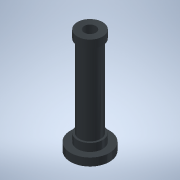
# Autodesk Inventor part: steering_stand_off_bush
Saved by Autodesk Inventor 2020 (Build 240168000, 168)
## iProperties
Created: 2015-12-07
Part Number: steering_stand_off_bush
Material: Hierro, gris
Document SubType Name: Modeling
Designer: MIGUEL ANGEL
Density: 7.15 g/cm^3
Appearance: Gris hierro
Author: MIGUEL ANGEL
Autodesk Inventor part; units mm, degrees
ref_plane "YZ Plane" through (0, 0, 0) normal (1, 0, 0) x (0, 1, 0)
ref_plane "XZ Plane" through (0, 0, 0) normal (0, 1, 0) x (-1, 0, 0)
ref_plane "XY Plane" through (0, 0, 0) normal (0, 0, 1) x (1, 0, 0)
sketch "Boceto1" plane through (0, 0, 0) normal (0, 0, 1) x (1, 0, 0)
  circle A0 centre (0, 0) radius 10
  dimension "d0" = 20
  constraints: 1 centre point, 1 coincident
  measures "d0" diameter of A0
extrude "Extrusión1" add sketch "Boceto1" along normal blind 4
sketch "Boceto2" plane through (0, 0, 4) normal (0, 0, 1) x (1, 0, 0)
  circle A0 centre (0, 0) radius 6.5
  dimension "d3" = 13
  constraints: 1 centre point, 1 coincident
  measures "d3" diameter of A0
extrude "Extrusión2" add sketch "Boceto2" along normal blind 50
sketch "Boceto3" plane through (0, 0, 0) normal (0, 1, 0) x (-1, 0, 0)
  line L0 (6.5, 50) -> (5.5, 50)
  line L1 (5.5, 50) -> (5.5, 8)
  line L2 (5.5, 8) -> (6.5, 8)
  line L3 (0, 30.7495) -> (0, -2.427)
  line L4 (10, 4) -> (-10, 4) projected
  line L5 (6.5, 4) -> (6.5, 54) projected
  point P0 (0, 0)
  dimension "d6" = 1
  dimension "d7" = 4
  dimension "d8" = 4
  constraints: 8 end point, 2 perpendicular, 2 point on line, 1 horizontal, 1 other
  measures "d6" distance of L0.start L0.end
  measures "d7" distance of L5.end L0.start
  measures "d8" distance of L5.start L2.end
revolve "Revolución1" cut sketch "Boceto3" angle 360 about axis through (0, 0, 30.7495) along (0, 0, -1)
sketch "Boceto4" plane through (0, 0, 54) normal (0, 0, 1) x (1, 0, 0)
  circle A0 centre (0, 0) radius 3
  dimension "d10" = 6
  constraints: 1 centre point, 1 coincident
  measures "d10" diameter of A0
extrude "Extrusión3" cut sketch "Boceto4" against normal blind 10
